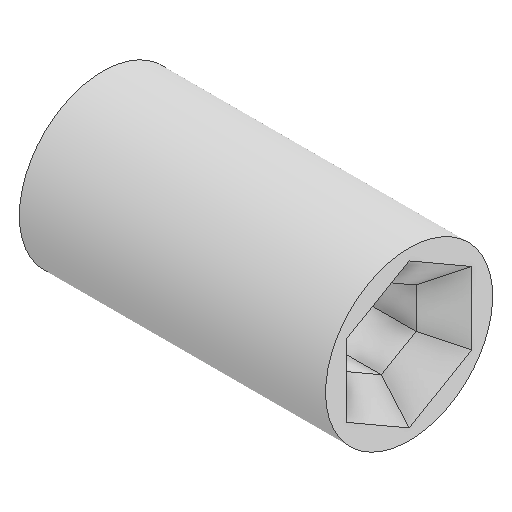
# Autodesk Inventor part: 40_XYZstage_micrometer_motorized_nema8_zadapter_m2.5nut
Saved by Autodesk Inventor 2024.1 (Build 281209000, 209)
## iProperties
Created: 2023-12-14
Part Number: 40_XYZstage_micrometer_motorized_nema8_zadapter_m2.5nut
Material: Generisch
Document SubType Name: Modeling
Designer: diederichbenedict
Density: 1 g/cm^3
Appearance: Vorgabe
Author: diederichbenedict
Autodesk Inventor part; units mm, degrees
ref_plane "YZ Plane" through (0, 0, 0) normal (1, 0, 0) x (0, 1, 0)
ref_plane "XZ Plane" through (0, 0, 0) normal (0, 1, 0) x (-1, 0, 0)
ref_plane "XY Plane" through (0, 0, 0) normal (0, 0, 1) x (1, 0, 0)
sketch "Skizze1" plane through (0, 0, 0) normal (1, 0, 0) x (0, 1, 0)
  circle A0 centre (0, 0) radius 3
  line L0 (1.4434, 0) -> (0.7217, -1.25)
  line L1 (0.7217, -1.25) -> (-0.7217, -1.25)
  line L2 (-0.7217, -1.25) -> (-1.4434, 0)
  line L3 (-1.4434, 0) -> (-0.7217, 1.25)
  line L4 (-0.7217, 1.25) -> (0.7217, 1.25)
  line L5 (0.7217, 1.25) -> (1.4434, 0)
  point P0 (0, -1.25)
  point P1 (0, 1.25)
  dimension "d0" = 6
  dimension "d1" = 2.5
  constraints: 12 end point, 2 coincident, 2 midpoint, 1 centre point, 13 other
  measures "d0" diameter of A0
  measures "d1" distance of point (0, -1.25) point (0, 1.25)
extrude "Extrusion1" add sketch "Skizze1" along normal blind 6
sketch "Skizze2" plane through (0, 0, 0) normal (-1, 0, 0) x (0, 0, 1)
  circle A0 centre (0, 0) radius 3 projected
  line L0 (0, 1.4434) -> (-1.25, 0.7217) projected
  line L1 (1.25, 0.7217) -> (0, 1.4434) projected
  line L2 (1.25, -0.7217) -> (1.25, 0.7217) projected
  line L3 (0, -1.4434) -> (1.25, -0.7217) projected
  line L4 (-1.25, -0.7217) -> (0, -1.4434) projected
  line L5 (-1.25, 0.7217) -> (-1.25, -0.7217) projected
  circle A1 centre (0, 0) radius 3
  constraints: 1 centre point, 1 coincident, 1 concentric
extrude "Extrusion2" add sketch "Skizze2" along normal blind 5 contours A0 | L1 L2 L3 L4 L5 L0
chamfer "Fase1" distance 1 angle 45 6 edges at (6, 1.0825, 0.625) (6, 1.0825, -0.625) (6, 0, -1.25) (6, -1.0825, -0.625) (6, -1.0825, 0.625) (6, 0, 1.25)
